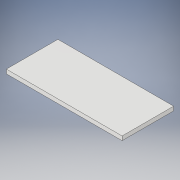
# Autodesk Inventor part: bepf_platforma_wypelnienie_polka_dolna
Saved by Autodesk Inventor 2017 (Build 210142000, 142)
## iProperties
Created: 2016-11-24
Part Number: bepf_platforma_wypelnienie_polka_dolna
Material: Tworzywo o ultrawysokiej masie cząsteczkowej, białe
Document SubType Name: Modeling
Designer: gagato
Mass: 72.6291 g
Surface Area: 287.04 cm^2
Volume: 77.265 cm^3
Density: 0.94 g/cm^3
Appearance: Gładki - biały
Author: gagato
Autodesk Inventor part; units mm, degrees
ref_plane "YZ Plane" through (0, 0, 0) normal (1, 0, 0) x (0, 1, 0)
ref_plane "XZ Plane" through (0, 0, 0) normal (0, 1, 0) x (-1, 0, 0)
ref_plane "XY Plane" through (0, 0, 0) normal (0, 0, 1) x (1, 0, 0)
sketch "Szkic1" plane through (0, 0, 0) normal (0, 1, 0) x (-1, 0, 0)
  line L0 (-85, -37.875) -> (85, -37.875)
  line L1 (85, -37.875) -> (85, 37.875)
  line L2 (85, 37.875) -> (-85, 37.875)
  line L3 (-85, 37.875) -> (-85, -37.875)
  line L4 (-85, -37.875) -> (85, 37.875) construction
  line L5 (85, -37.875) -> (-85, 37.875) construction
  point P0 (0, 0)
  dimension "d0" = 170
  dimension "d1" = 75.75
  constraints: 12 end point, 2 midpoint, 2 parallel, 1 horizontal, 1 perpendicular
  measures "d0" distance of L2.end L1.end
  measures "d1" distance of L1.end L0.end
extrude "Wyciągnięcie proste1" add sketch "Szkic1" along normal mid plane 6
